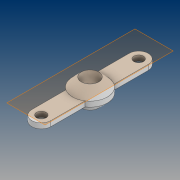
# Autodesk Inventor part: 12_Thong_lo_xo
Saved by Autodesk Inventor 2021 (Build 250183000, 183)
## iProperties
Created: 2024-04-04
Part Number: 12_Thong_lo_xo
Material: Generic
Document SubType Name: Modeling
Designer: Admin
Density: 1 g/cm^3
Appearance: Default
Author: Admin
Autodesk Inventor part; units mm, degrees
ref_plane "YZ Plane" through (0, 0, 0) normal (1, 0, 0) x (0, 1, 0)
ref_plane "XZ Plane" through (0, 0, 0) normal (0, 1, 0) x (-1, 0, 0)
ref_plane "XY Plane" through (0, 0, 0) normal (0, 0, 1) x (1, 0, 0)
sketch "Sketch1" plane through (0, 0, 0) normal (0, 1, 0) x (-1, 0, 0)
  circle A0 centre (0, 0) radius 10
  line L0 (0, 28) -> (0, -28) construction
  line L1 (-5.5, 28) -> (-5.5, -28)
  line L2 (5.5, -28) -> (5.5, 28)
  arc A1 (5.5, 28) -> (-5.5, 28) centre (0, 28) ccw
  arc A2 (-5.5, -28) -> (5.5, -28) centre (0, -28) ccw
  circle A3 centre (0, 0) radius 5
  circle A4 centre (0, 28) radius 2.75
  circle A5 centre (0, -28) radius 2.75
  point P0 (-5.5, 8.3516)
  point P1 (-5.5, -8.3516)
  point P2 (5.5, -8.3516)
  point P3 (5.5, 8.3516)
  dimension "d0" = 56
  dimension "d1" = 20
  dimension "d2" = 10
  dimension "d3" = 5.5
  dimension "d4" = 5.5
  constraints: 8 end point, 6 centre point, 4 coincident, 4 point on circle, 4 tangent, 1 equal radius, 1 midpoint, 1 parallel, 1 vertical
  measures "d0" distance of L0.start L0.end
  measures "d1" diameter of A0
  measures "d2" diameter of A3
  measures "d3" radius of A2
  measures "d4" diameter of A5
extrude "Extrusion1" add sketch "Sketch1" along normal blind 1.5
ref_plane "Work Plane1" through (0, 6.5, 0) normal (0, 1, 0) x (1, 0, 0)
sketch "Sketch4" plane through (0, 1.5, 0) normal (0, 1, 0) x (1, 0, 0)
  arc A0 (5.5, -8.3516) -> (5.5, 8.3516) centre (0, 0) ccw projected
  circle A1 centre (0, 0) radius 10
  constraints: 1 centre point, 1 coincident
sketch "Sketch2" plane through (0, 6.5, 0) normal (0, 1, 0) x (1, 0, 0)
  circle A0 centre (0, 0) radius 5 projected
  circle A1 centre (0, 0) radius 5
  constraints: 1 centre point, 1 coincident, 1 concentric
loft "Loft2" add profiles "Sketch2", "Sketch4"
sketch "Sketch3" plane through (0, 0, 0) normal (0, -1, 0) x (1, 0, 0)
  circle A0 centre (0, 0) radius 5 projected
  circle A1 centre (0, 28) radius 2.75 projected
  circle A2 centre (0, -28) radius 2.75 projected
extrude "Extrusion2" cut sketch "Sketch3" against normal through all
mirror "Mirror1" about plane through (0, 0, 0) normal (0, -1, 0) of "Extrusion1", "Loft2", "Extrusion2"
body "Solid1"
